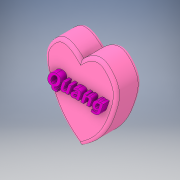
# Autodesk Inventor part: heart
Saved by Autodesk Inventor 2017 (Build 210142000, 142)
## iProperties
Created: 2019-02-08
Part Number: heart
Material: Generic
Document SubType Name: Modeling
Designer: qthuynh
Density: 1 g/cm^3
Appearance: Default
Author: qthuynh
Autodesk Inventor part; units mm, degrees
ref_plane "YZ Plane" through (0, 0, 0) normal (1, 0, 0) x (0, 1, 0)
ref_plane "XZ Plane" through (0, 0, 0) normal (0, 1, 0) x (-1, 0, 0)
ref_plane "XY Plane" through (0, 0, 0) normal (0, 0, 1) x (1, 0, 0)
sketch "Sketch1" plane through (0, 0, 0) normal (0, 0, 1) x (1, 0, 0)
  line L0 (0, 0) -> (0, 76.2)
  line L1 (0, 76.2) -> (-6.8414, 83.2449) construction
  line L2 (-6.8414, 83.2449) -> (-19.997, 89.9831) construction
  line L3 (-19.997, 89.9831) -> (-29.623, 80.0362) construction
  line L4 (-29.623, 80.0362) -> (-41.4951, 64.3137) construction
  line L5 (-41.4951, 64.3137) -> (-32.8317, 43.4574) construction
  line L6 (-32.8317, 43.4574) -> (-22.2431, 14.5793) construction
  line L7 (-22.2431, 14.5793) -> (0, 0) construction
  spline S0 degree 4 poles (0, 76.2) (-6.8414, 83.2449) (-19.997, 89.9831) (-29.623, 80.0362) (-41.4951, 64.3137) (-32.8317, 43.4574) (-22.2431, 14.5793) (0, 0) knots 1 1 1 1 1 2 3 4 5 5 5 5 5
  dimension "d0" = 76.2
  constraints: 2 end point, 1 vertical, 3 other
  measures "d0" distance of L0.start L0.end
extrude "Extrusion1" add sketch "Sketch1" along normal blind 25.4
mirror "Mirror1" about plane through (0, 0, 0) normal (1, 0, 0) of "Extrusion1"
fillet "Fillet1" radius 3.175 4 edges at (-34.543, 71.5689, 25.4) (34.543, 71.5689, 25.4) (-34.543, 71.5689, 0) (34.543, 71.5689, 0)
sketch "Sketch2" plane through (0, 0, 25.4) normal (0, 0, 1) x (1, 0, 0)
  line L0 (-29.8365, 58.3408) -> (-8.2127, 58.3408) construction
  line L1 (-8.2127, 58.3408) -> (-8.2127, 65.6431) construction
  line L2 (-8.2127, 65.6431) -> (-29.8365, 65.6431) construction
  line L3 (-29.8365, 65.6431) -> (-29.8365, 58.3408) construction
  spline S0 degree 2 poles (-18.1245, 42.0181) (-18.6803, 41.8946) (-19.7506, 41.7711) (-20.8518, 41.7711) knots 0 0 0 1 2 2 2
  spline S1 degree 2 poles (-20.8518, 41.7711) (-21.8501, 41.7711) (-23.0851, 42.2754) (-23.4042, 42.7386) knots 0 0 0 1 2 2 2
  spline S2 degree 2 poles (-23.4042, 42.7386) (-23.7129, 43.1914) (-23.7644, 44.4264) (-23.5483, 45.1468) knots 0 0 0 1 2 2 2
  spline S3 degree 2 poles (-23.5483, 45.1468) (-26.2035, 45.2703) (-28.1075, 48.7592) (-27.0989, 51.7232) knots 0 0 0 1 2 2 2
  spline S4 degree 2 poles (-27.0989, 51.7232) (-26.0594, 54.7799) (-21.5825, 58.3408) (-18.7111, 58.3408) knots 0 0 0 1 2 2 2
  spline S5 degree 2 poles (-18.7111, 58.3408) (-15.8397, 58.3408) (-13.7608, 54.8005) (-14.8003, 51.7232) knots 0 0 0 1 2 2 2
  spline S6 degree 2 poles (-14.8003, 51.7232) (-15.5619, 49.4796) (-18.5259, 46.2686) (-20.4607, 45.5894) knots 0 0 0 1 2 2 2
  spline S7 degree 2 poles (-20.4607, 45.5894) (-20.7592, 44.6528) (-20.2137, 43.9427) (-19.2154, 43.9427) knots 0 0 0 1 2 2 2
  spline S8 degree 2 poles (-19.2154, 43.9427) (-18.8346, 43.9427) (-17.8981, 44.1691) (-17.6717, 44.272) knots 0 0 0 1 2 2 2
  line L4 (-17.6717, 44.272) -> (-17.3526, 44.272)
  line L5 (-17.3526, 44.272) -> (-18.1245, 42.0181)
  spline S9 degree 2 poles (-20.0388, 48.5122) (-19.4419, 49.068) (-18.495, 50.5397) (-18.0936, 51.7335) knots 0 0 0 1 2 2 2
  spline S10 degree 2 poles (-18.0936, 51.7335) (-17.7128, 52.8656) (-17.6305, 54.4608) (-17.8569, 54.9754) knots 0 0 0 1 2 2 2
  spline S11 degree 2 poles (-17.8569, 54.9754) (-18.0833, 55.49) (-18.9581, 55.9428) (-19.5139, 55.9428) knots 0 0 0 1 2 2 2
  spline S12 degree 2 poles (-19.5139, 55.9428) (-20.1005, 55.9428) (-21.2017, 55.5209) (-21.8192, 54.9857) knots 0 0 0 1 2 2 2
  spline S13 degree 2 poles (-21.8192, 54.9857) (-22.3853, 54.4917) (-23.4248, 52.8553) (-23.8055, 51.7232) knots 0 0 0 1 2 2 2
  spline S14 degree 2 poles (-23.8055, 51.7232) (-24.2069, 50.5603) (-24.2687, 49.0165) (-24.0423, 48.4916) knots 0 0 0 1 2 2 2
  spline S15 degree 2 poles (-24.0423, 48.4916) (-23.8158, 47.9668) (-22.9307, 47.5139) (-22.375, 47.5139) knots 0 0 0 1 2 2 2
  spline S16 degree 2 poles (-22.375, 47.5139) (-21.8192, 47.5139) (-20.5945, 47.9976) (-20.0388, 48.5122) knots 0 0 0 1 2 2 2
  line L6 (-6.3508, 45.3732) -> (-9.3354, 45.3732)
  line L7 (-9.3354, 45.3732) -> (-8.9752, 46.4333)
  spline S17 degree 2 poles (-8.9752, 46.4333) (-9.9735, 45.7849) (-11.4966, 45.1057) (-12.392, 45.1057) knots 0 0 0 1 2 2 2
  spline S18 degree 2 poles (-12.392, 45.1057) (-13.8123, 45.1057) (-14.79, 46.9067) (-14.1828, 48.7181) knots 0 0 0 1 2 2 2
  line L8 (-14.1828, 48.7181) -> (-12.0627, 54.9548)
  line L9 (-12.0627, 54.9548) -> (-9.0575, 54.9548)
  line L10 (-9.0575, 54.9548) -> (-10.6733, 50.2001)
  spline S19 degree 2 poles (-10.6733, 50.2001) (-10.9203, 49.4591) (-11.1673, 48.5122) (-11.1261, 48.1932) knots 0 0 0 1 2 2 2
  spline S20 degree 2 poles (-11.1261, 48.1932) (-11.0953, 47.8947) (-10.6321, 47.586) (-10.1175, 47.586) knots 0 0 0 1 2 2 2
  spline S21 degree 2 poles (-10.1175, 47.586) (-9.8088, 47.586) (-8.8414, 47.8947) (-8.3885, 48.1623) knots 0 0 0 1 2 2 2
  line L11 (-8.3885, 48.1623) -> (-6.0832, 54.9548)
  line L12 (-6.0832, 54.9548) -> (-3.0986, 54.9548)
  line L13 (-3.0986, 54.9548) -> (-6.3508, 45.3732)
  spline S22 degree 2 poles (1.5636, 46.3921) (1.1622, 46.1348) (0.5344, 45.7232) (0.061, 45.5173) knots 0 0 0 1 2 2 2
  spline S23 degree 2 poles (0.061, 45.5173) (-0.4124, 45.3218) (-1.2358, 45.1159) (-1.9253, 45.1159) knots 0 0 0 1 2 2 2
  spline S24 degree 2 poles (-1.9253, 45.1159) (-3.1912, 45.1159) (-4.2924, 46.8244) (-3.8499, 48.1211) knots 0 0 0 1 2 2 2
  spline S25 degree 2 poles (-3.8499, 48.1211) (-3.4897, 49.1812) (-2.1929, 50.4985) (-1.2564, 50.8793) knots 0 0 0 1 2 2 2
  spline S26 degree 2 poles (-1.2564, 50.8793) (-0.3198, 51.2704) (2.037, 51.5792) (3.3646, 51.6615) knots 0 0 0 1 2 2 2
  line L14 (3.3646, 51.6615) -> (3.3852, 51.7129)
  spline S27 degree 2 poles (3.3852, 51.7129) (3.6528, 52.5054) (2.6957, 53.1126) (1.5224, 53.1126) knots 0 0 0 1 2 2 2
  spline S28 degree 2 poles (1.5224, 53.1126) (0.9975, 53.1126) (-0.5565, 52.7318) (-1.3284, 52.4334) knots 0 0 0 1 2 2 2
  line L15 (-1.3284, 52.4334) -> (-1.5857, 52.4334)
  line L16 (-1.5857, 52.4334) -> (-0.8035, 54.749)
  spline S29 degree 2 poles (-0.8035, 54.749) (-0.3095, 54.8725) (1.79, 55.2224) (2.7883, 55.2224) knots 0 0 0 1 2 2 2
  spline S30 degree 2 poles (2.7883, 55.2224) (5.2686, 55.2224) (6.9667, 53.5758) (6.3904, 51.8879) knots 0 0 0 1 2 2 2
  line L17 (6.3904, 51.8879) -> (4.1777, 45.3732)
  line L18 (4.1777, 45.3732) -> (1.2137, 45.3732)
  line L19 (1.2137, 45.3732) -> (1.5636, 46.3921)
  line L20 (2.0679, 47.8741) -> (2.7368, 49.8604)
  spline S31 degree 2 poles (2.7368, 49.8604) (1.9547, 49.7884) (0.9769, 49.6752) (0.4624, 49.5105) knots 0 0 0 1 2 2 2
  spline S32 degree 2 poles (0.4624, 49.5105) (0.0301, 49.3767) (-0.5977, 48.821) (-0.7521, 48.3681) knots 0 0 0 1 2 2 2
  spline S33 degree 2 poles (-0.7521, 48.3681) (-0.9785, 47.6992) (-0.4227, 47.1949) (0.2874, 47.1949) knots 0 0 0 1 2 2 2
  spline S34 degree 2 poles (0.2874, 47.1949) (0.6785, 47.1949) (1.6253, 47.5551) (2.0679, 47.8741) knots 0 0 0 1 2 2 2
  line L21 (15.3545, 45.3732) -> (12.3493, 45.3732)
  line L22 (12.3493, 45.3732) -> (13.9651, 50.1177)
  spline S35 degree 2 poles (13.9651, 50.1177) (14.1607, 50.7044) (14.4591, 51.857) (14.4282, 52.1246) knots 0 0 0 1 2 2 2
  spline S36 degree 2 poles (14.4282, 52.1246) (14.3768, 52.454) (13.9034, 52.7318) (13.4094, 52.7318) knots 0 0 0 1 2 2 2
  spline S37 degree 2 poles (13.4094, 52.7318) (13.0492, 52.7318) (12.2052, 52.454) (11.6804, 52.1555) knots 0 0 0 1 2 2 2
  line L23 (11.6804, 52.1555) -> (9.375, 45.3732)
  line L24 (9.375, 45.3732) -> (6.3904, 45.3732)
  line L25 (6.3904, 45.3732) -> (9.6426, 54.9548)
  line L26 (9.6426, 54.9548) -> (12.6272, 54.9548)
  line L27 (12.6272, 54.9548) -> (12.267, 53.8948)
  spline S38 degree 2 poles (12.267, 53.8948) (13.2138, 54.5123) (14.8399, 55.2121) (15.6838, 55.2121) knots 0 0 0 1 2 2 2
  spline S39 degree 2 poles (15.6838, 55.2121) (17.1453, 55.2121) (18.0715, 53.3596) (17.4746, 51.61) knots 0 0 0 1 2 2 2
  line L28 (17.4746, 51.61) -> (15.3545, 45.3732)
  spline S40 degree 2 poles (26.6445, 46.4745) (26.202, 45.1468) (24.8023, 43.284) (23.9584, 42.7694) knots 0 0 0 1 2 2 2
  spline S41 degree 2 poles (23.9584, 42.7694) (23.1145, 42.2446) (21.0973, 41.7711) (19.9652, 41.7711) knots 0 0 0 1 2 2 2
  spline S42 degree 2 poles (19.9652, 41.7711) (19.0081, 41.7711) (17.382, 42.0181) (16.8056, 42.1828) knots 0 0 0 1 2 2 2
  line L29 (16.8056, 42.1828) -> (17.6187, 44.5808)
  line L30 (17.6187, 44.5808) -> (17.9686, 44.5808)
  spline S43 degree 2 poles (17.9686, 44.5808) (18.1641, 44.4984) (18.6993, 44.2926) (18.9772, 44.2103) knots 0 0 0 1 2 2 2
  spline S44 degree 2 poles (18.9772, 44.2103) (19.3065, 44.1176) (19.9652, 43.9941) (20.3357, 43.9941) knots 0 0 0 1 2 2 2
  spline S45 degree 2 poles (20.3357, 43.9941) (21.087, 43.9941) (22.2088, 44.3029) (22.569, 44.5911) knots 0 0 0 1 2 2 2
  spline S46 degree 2 poles (22.569, 44.5911) (22.9189, 44.8895) (23.4026, 45.6923) (23.6085, 46.3098) knots 0 0 0 1 2 2 2
  line L31 (23.6085, 46.3098) -> (23.6702, 46.4847)
  spline S47 degree 2 poles (23.6702, 46.4847) (23.0116, 46.0422) (21.509, 45.507) (20.8091, 45.507) knots 0 0 0 1 2 2 2
  spline S48 degree 2 poles (20.8091, 45.507) (18.9566, 45.507) (17.7525, 47.9256) (18.5964, 50.4059) knots 0 0 0 1 2 2 2
  spline S49 degree 2 poles (18.5964, 50.4059) (18.9772, 51.5277) (20.2122, 53.3185) (20.9841, 53.9463) knots 0 0 0 1 2 2 2
  spline S50 degree 2 poles (20.9841, 53.9463) (21.7148, 54.5535) (23.4335, 55.2121) (24.2466, 55.2121) knots 0 0 0 1 2 2 2
  spline S51 degree 2 poles (24.2466, 55.2121) (24.9773, 55.2121) (26.0167, 54.8416) (26.3872, 54.5329) knots 0 0 0 1 2 2 2
  line L32 (26.3872, 54.5329) -> (26.6445, 54.9548)
  line L33 (26.6445, 54.9548) -> (29.5262, 54.9548)
  line L34 (29.5262, 54.9548) -> (26.6445, 46.4745)
  line L35 (24.3186, 48.3887) -> (25.7903, 52.7318)
  spline S52 degree 2 poles (25.7903, 52.7318) (25.6051, 52.8347) (24.9979, 52.9685) (24.6788, 52.9685) knots 0 0 0 1 2 2 2
  spline S53 degree 2 poles (24.6788, 52.9685) (23.6085, 52.9685) (22.0544, 51.5792) (21.6325, 50.3339) knots 0 0 0 1 2 2 2
  spline S54 degree 2 poles (21.6325, 50.3339) (21.4163, 49.7164) (21.2928, 48.8518) (21.3957, 48.5225) knots 0 0 0 1 2 2 2
  spline S55 degree 2 poles (21.3957, 48.5225) (21.4987, 48.1932) (22.075, 47.8638) (22.6102, 47.8638) knots 0 0 0 1 2 2 2
  spline S56 degree 2 poles (22.6102, 47.8638) (23.0116, 47.8638) (23.8761, 48.1417) (24.3186, 48.3887) knots 0 0 0 1 2 2 2
  point P0 (0, 0)
  constraints: 2 other
extrude "Extrusion2" add sketch "Sketch2" along normal blind 6.35
body "Solid1"
